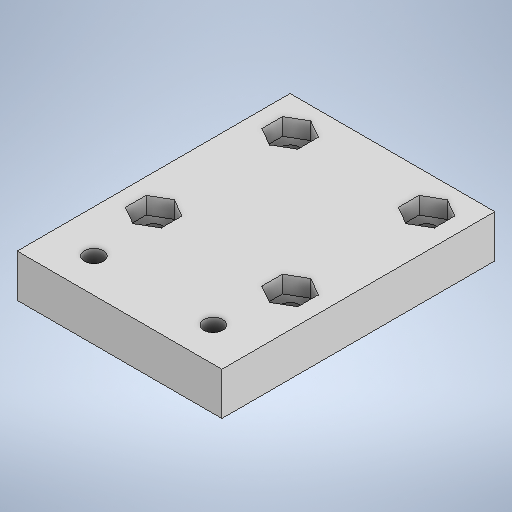
# Autodesk Inventor part: robot_left
Saved by Autodesk Inventor 2025.1 (Build 291241000, 241)
## iProperties
Created: 2024-11-20
Part Number: robot_left
Material: 일반
Document SubType Name: Modeling
Designer: goode
Density: 1 g/cm^3
Appearance: 기본값
Author: goode
Autodesk Inventor part; units mm, degrees
ref_plane "YZ Plane" through (0, 0, 0) normal (1, 0, 0) x (0, 1, 0)
ref_plane "XZ Plane" through (0, 0, 0) normal (0, 1, 0) x (-1, 0, 0)
ref_plane "XY Plane" through (0, 0, 0) normal (0, 0, 1) x (1, 0, 0)
sketch "스케치1" plane through (0, 0, 0) normal (0, 1, 0) x (-1, 0, 0)
  line L0 (0, 0) -> (24, 0)
  line L1 (24, 0) -> (24, -24)
  line L2 (24, -24) -> (0, -24)
  line L3 (0, -24) -> (0, 0)
  circle A0 centre (4, -4) radius 1.1
  circle A1 centre (4, -4) radius 2.1
  line L4 (1.9, -4) -> (4, -4)
  line L5 (1.9, -2.7876) -> (4, -1.5751)
  line L6 (4, -1.5751) -> (6.1, -2.7876)
  line L7 (6.1, -2.7876) -> (6.1, -5.2124)
  line L8 (6.1, -5.2124) -> (4, -6.4249)
  line L9 (4, -6.4249) -> (1.9, -5.2124)
  line L10 (1.9, -5.2124) -> (1.9, -2.7876)
  circle A2 centre (4, -20) radius 1.1
  circle A3 centre (4, -20) radius 2.1
  line L11 (1.9, -20) -> (4, -20)
  line L12 (1.9, -18.7876) -> (4, -17.5751)
  line L13 (4, -17.5751) -> (6.1, -18.7876)
  line L14 (6.1, -18.7876) -> (6.1, -21.2124)
  line L15 (6.1, -21.2124) -> (4, -22.4249)
  line L16 (4, -22.4249) -> (1.9, -21.2124)
  line L17 (1.9, -21.2124) -> (1.9, -18.7876)
  circle A4 centre (20, -4) radius 1.1
  circle A5 centre (20, -4) radius 2.1
  line L18 (17.9, -4) -> (20, -4)
  line L19 (17.9, -2.7876) -> (20, -1.5751)
  line L20 (20, -1.5751) -> (22.1, -2.7876)
  line L21 (22.1, -2.7876) -> (22.1, -5.2124)
  line L22 (22.1, -5.2124) -> (20, -6.4249)
  line L23 (20, -6.4249) -> (17.9, -5.2124)
  line L24 (17.9, -5.2124) -> (17.9, -2.7876)
  circle A6 centre (20, -20) radius 1.1
  circle A7 centre (20, -20) radius 2.1
  line L25 (17.9, -20) -> (20, -20)
  line L26 (17.9, -18.7876) -> (20, -17.5751)
  line L27 (20, -17.5751) -> (22.1, -18.7876)
  line L28 (22.1, -18.7876) -> (22.1, -21.2124)
  line L29 (22.1, -21.2124) -> (20, -22.4249)
  line L30 (20, -22.4249) -> (17.9, -21.2124)
  line L31 (17.9, -21.2124) -> (17.9, -18.7876)
  line L32 (12, 0) -> (12, 4)
  line L33 (12, 4) -> (19, 4)
  line L34 (12, 4) -> (5, 4)
  dimension "d3" = 4.2
  dimension "d0" = 24
  dimension "d1" = 24
  dimension "d2" = 2.2
  dimension "d6" = 16
  dimension "d9" = 16
  dimension "d12" = 4
  dimension "d13" = 7
  dimension "d14" = 7
  constraints: 70 end point, 8 coincident, 6 horizontal, 4 centre point, 4 horizontal alignment, 3 vertical, 2 midpoint, 2 parallel, 2 perpendicular, 75 other
  measures "d0" distance of L1.end L2.end
  measures "d1" distance of L0.end L1.end
  measures "d2" diameter of A0
  measures "d6" distance of A0.centre A2.centre
  measures "d9" distance of A0.centre A4.centre
  measures "d12" distance of L32.start L32.end
  measures "d13" distance of L32.end L33.end
  measures "d14" distance of L32.end L34.end
extrude "돌출1" add sketch "스케치1" against normal blind 5 contours L0 L1 L2 L3 | A0 | A1 | A1 L9 L10 | L10 L5 A1 | L5 L6 A1 | A1 L8 L9 | L6 L7 A1 | A1 L7 L8 | A2 | A3 | A3 L16 L17 | L17 L12 A3 | L12 L13 A3 | A3 L15 L16 | L13 L14 A3 | A3 L14 L15 | A4 | A5 | A5 L23 L24 | L24 L19 A5 | L19 L20 A5 | A5 L22 L23 | L20 L21 A5 | A5 L21 L22 | A6 | A7 | A7 L30 L31 | L31 L26 A7 | L26 L27 A7 | A7 L29 L30 | L27 L28 A7 | A7 L28 L29
extrude "돌출2" cut sketch "스케치1" against normal blind 2 contours A0 | A1 | A1 L9 L10 | L10 L5 A1 | L5 L6 A1 | A1 L8 L9 | L6 L7 A1 | A1 L7 L8 | A2 | A3 | A3 L16 L17 | L17 L12 A3 | L12 L13 A3 | A3 L15 L16 | L13 L14 A3 | A3 L14 L15 | A4 | A5 | A5 L23 L24 | L24 L19 A5 | L19 L20 A5 | A5 L22 L23 | L20 L21 A5 | A5 L21 L22 | A6 | A7 | A7 L30 L31 | L31 L26 A7 | L26 L27 A7 | A7 L29 L30 | L27 L28 A7 | A7 L28 L29
extrude "돌출3" cut sketch "스케치1" against normal blind 5 contours A0 | A2 | A4 | A6
sketch "스케치2" plane through (0, 0, 0) normal (0, 1, 0) x (1, 0, 0)
  line L0 (0, 0) -> (-24, 0)
  line L1 (-24, 0) -> (-24, -8)
  line L2 (-24, -8) -> (0, -8)
  line L3 (0, -8) -> (0, 0)
  dimension "d21" = 8
  constraints: 8 end point, 2 parallel, 1 horizontal, 1 perpendicular
  measures "d21" distance of L1.end L0.end
extrude "돌출4" add sketch "스케치2" against normal blind 5
sketch "스케치3" plane through (0, -5, 0) normal (0, -1, 0) x (1, 0, 0)
  line L0 (0, 0) -> (-12, 0)
  line L1 (-12, 0) -> (-12, 4)
  line L2 (-12, 4) -> (-5, 4)
  line L3 (-12, 4) -> (-19, 4)
  circle A0 centre (-5, 4) radius 1.1
  circle A1 centre (-5, 4) radius 2.1
  circle A2 centre (-19, 4) radius 1.1
  circle A3 centre (-19, 4) radius 2.1
  line L4 (-2.9, 2.7876) -> (-5, 1.5751)
  line L5 (-5, 1.5751) -> (-7.1, 2.7876)
  line L6 (-7.1, 2.7876) -> (-7.1, 5.2124)
  line L7 (-7.1, 5.2124) -> (-5, 6.4249)
  line L8 (-5, 6.4249) -> (-2.9, 5.2124)
  line L9 (-2.9, 5.2124) -> (-2.9, 2.7876)
  line L10 (-21.1, 5.2124) -> (-19, 6.4249)
  line L11 (-19, 6.4249) -> (-16.9, 5.2124)
  line L12 (-16.9, 5.2124) -> (-16.9, 2.7876)
  line L13 (-16.9, 2.7876) -> (-19, 1.5751)
  line L14 (-19, 1.5751) -> (-21.1, 2.7876)
  line L15 (-21.1, 2.7876) -> (-21.1, 5.2124)
  point P0 (-2.9, 4)
  point P1 (-21.1, 4)
  dimension "d29" = 4.2
  dimension "d31" = 4.2
  dimension "d24" = 12
  dimension "d25" = 4
  dimension "d26" = 7
  dimension "d27" = 7
  dimension "d28" = 2.2
  dimension "d30" = 2.2
  constraints: 32 end point, 6 coincident, 2 centre point, 2 horizontal, 2 horizontal alignment, 2 midpoint, 2 perpendicular, 1 point on line, 30 other
  measures "d24" distance of L0.start L0.end
  measures "d25" distance of L0.end L1.end
  measures "d26" distance of L1.end L2.end
  measures "d27" distance of L1.end L3.end
  measures "d28" diameter of A0
  measures "d30" diameter of A2
extrude "돌출5" cut sketch "스케치3" against normal blind 2 contours L6 L7 A1 | A0 | A1 | A1 L5 L6 | L12 L13 A3 | A2 | A3 | A3 L11 L12 | L7 L8 A1 | A1 L4 L5 | A3 L10 L11 | L13 L14 A3 | L8 L9 A1 | A1 L9 L4 | A3 L15 L10 | L14 L15 A3
extrude "돌출6" cut sketch "스케치3" against normal blind 5 contours A0 | A2
